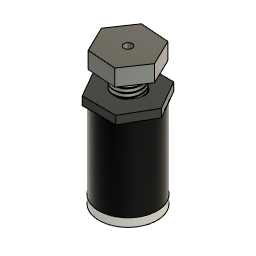
Electrode holder v2 (Autodesk Fusion 360 design; units mm, degrees)
Autodesk Fusion 360 part; units mm, degrees
note: some values were not read from the file. Set by a fixed rule: which face or edge a step refers to.
sketch "Sketch1" plane through (0, 0, 0) normal (0, 0, 1) x (1, 0, 0)
  circle A0 centre (0, 0) radius 5
  circle A1 centre (0, 0) radius 7
  dimension "d1" = 10
  dimension "d2" = 14
  constraint coincident A0.centre A1.centre
  constraint concentric A0 A1
  measures "d1" diameter of A0
  measures "d2" diameter of A1
extrude "Extrude1" add sketch "Sketch1" along normal blind 2 makes body 1
ref_plane "WorkPlane1" through (0, 0, 2.1) normal (0, 0, 1) x (1, 0, 0)
sketch "Sketch2" plane through (0, 0, 2.1) normal (0, 0, 1) x (1, 0, 0)
  circle A0 centre (0, 0) radius 5
  circle A1 centre (0, 0) radius 7
  dimension "d6" = 10
  dimension "d7" = 14
  constraint coincident A0.centre A1.centre
  constraint concentric A0 A1
  measures "d6" diameter of A0
  measures "d7" diameter of A1
extrude "Extrude2" add sketch "Sketch2" along normal blind 10 separate body makes body 2
sketch "Sketch3" plane through (0, 0, 0) normal (0, 0, -1) x (1, 0, 0)
  circle A0 centre (0, 0) radius 5
  circle A1 centre (0, 0) radius 7
  circle A2 centre (0, 0) radius 5
  circle A3 centre (0, 0) radius 4.5
  dimension "d10" = 9
  constraint coincident A0.centre A1.centre
  measures "d10" diameter of A3
extrude "Extrude3" add sketch "Sketch3" against normal blind 5.5 separate body contours A0 A2 makes body 3
combine "Combine1" operation add target body 3 tool bodies 1
sketch "Sketch4" plane through (0, 0, 12.1) normal (0, 0, 1) x (-1, 0, 0)
  circle A0 centre (0, 0) radius 5
  circle A1 centre (0, 0) radius 7
  circle A2 centre (0, 0) radius 4.5
  dimension "d13" = 9
  constraint coincident A0.centre A1.centre
  measures "d13" diameter of A2
extrude "Extrude4" add sketch "Sketch4" against normal blind 6.5 contours A0 bodies 2
sketch "Sketch5" plane through (0, 0, 12.1) normal (0, 0, 1) x (-1, 0, 0)
  circle A0 centre (0, 0) radius 4.5
  circle A1 centre (0, 0) radius 7
  line L0 (0, 0) -> (0, 4.5)
  circle A2 centre (0, 4.5) radius 1
  dimension "d16" = 2
  constraint coincident A0.centre A1.centre
  constraint coincident A0 L0.end
  constraint vertical L0
  constraint coincident L0.end A2.centre
  measures "d16" diameter of A2
extrude "Extrude5" cut sketch "Sketch5" against normal blind 8 contours A0 A2 picked at (-0.226, 4.8088) bodies 2
extrude "Extrude6" add 1 faces at (2.7671, -5.493, 12.1) along direction (0, 0, 1) blind 10 on bodies 2 bodies 2
sketch "Sketch6" plane through (0, 0, 0) normal (1, 0, 0) x (0, 1, 0)
  line L0 (-4.5, 5.5) -> (4.5, 5.5)
  line L1 (4.5, 0) -> (-4.5, 0)
  line L2 (-4.5, 0) -> (-4.5, 23.0015) construction
  circle A0 centre (-4.5, 8) radius 1
  circle A1 centre (-4.5, 12) radius 1
  circle A2 centre (-4.5, 16) radius 1
  circle A3 centre (-4.5, 20) radius 1
  dimension "d21" = 2
  dimension "d22" = 8
  dimension "d23" = 2
  dimension "d24" = 2
  dimension "d25" = 2
  dimension "d27" = 4
  dimension "d28" = 4
  dimension "d29" = 4
  constraint coincident L1.end L2.start
  constraint perpendicular L1 L2
  constraint coincident L2 A0.centre
  constraint coincident L2 A1.centre
  constraint coincident L2 A2.centre
  constraint coincident L2 A3.centre
  measures "d21" diameter of A0
  measures "d22" distance of L1.end A0.centre
  measures "d23" diameter of A1
  measures "d24" diameter of A2
  measures "d25" diameter of A3
  measures "d27" distance of A0.centre A1.centre
  measures "d28" distance of A1.centre A2.centre
  measures "d29" distance of A2.centre A3.centre
revolve "Revolve1" cut sketch "Sketch6" angle 40 about axis through (0, 0, 1.75) along (0, 0, -1) bodies 2
mirror "Mirror1" about plane through (0, 0, 0) normal (0, 1, 0) of "Extrude5"
extrude "Extrude7" cut 1 faces at (0, 5.1605, 4.1) along direction (0, 0, 1) blind 26.5 on bodies 2 bodies 2
ref_plane "WorkPlane2" through (0, 0, 12.125) normal (0.34202, 0.939693, 0) x (0, 0, 1)
mirror "Mirror2" about plane through (0, 0, 12.125) normal (0.34202, 0.939693, 0) of "Revolve1"
sketch "Sketch7" plane through (0, 0, 22.1) normal (0, 0, 1) x (-1, 0, 0)
  arc A0 (-0.9091, -4.9167) -> (0.9091, -4.9167) centre (0, -4.5) ccw
  arc A1 (0.9938, 4.3889) -> (-0.9938, 4.3889) centre (0, 4.5) ccw
  arc A2 (-0.9938, 4.3889) -> (0.9938, 4.3889) centre (0, 0) ccw
  circle A3 centre (0, 0) radius 7
  arc A4 (-0.9091, -4.9167) -> (0.9091, -4.9167) centre (0, 0) ccw
ref_plane "WorkPlane3" through (0, 0, 23.1) normal (0, 0, 1) x (-1, 0, 0)
sketch "Sketch8" plane through (0, 0, 23.1) normal (0, 0, 1) x (1, 0, 0)
  circle A0 centre (0, 0) radius 4.4
  circle A1 centre (0, 0) radius 2.5
  dimension "d40" = 8.8
  dimension "d43" = 5
  constraint coincident A0.centre A1.centre
  measures "d40" diameter of A0
  measures "d43" diameter of A1
extrude "Extrude9" add sketch "Sketch8" along normal blind 2 separate body makes body 4
sketch "Sketch9" plane through (0, 0, 0) normal (1, 0, 0) x (0, 1, 0)
  line L0 (4.4, 25.1) -> (-4.4, 25.1)
  line L1 (4.4, 23.1) -> (-4.4, 23.1)
  line L2 (-4.4, 25.1) -> (-4.4, 23.1) construction
  line L3 (4.4, 25.1) -> (4.4, 23.1) construction
  circle A0 centre (-4.4, 24.1) radius 1
  circle A1 centre (4.4, 24.1) radius 1
  line L4 (-4.4, 25.1) -> (-4.4, 23.1)
  line L5 (4.4, 25.1) -> (4.4, 23.1)
  constraint coincident L0.end L2.start
  constraint coincident L1.end L2.end
  constraint coincident L0.start L3.start
  constraint coincident L1.start L3.end
  constraint midpoint L2 A0.centre
  constraint coincident L1.end A0
  constraint midpoint L3 A1.centre
  constraint coincident L0.start A1
revolve "Revolve2" add sketch "Sketch9" angle 360 about axis through (0, 4.4, 25.1) along (0, 0, -1) contours A1 L5 picked at (4.6804, 24.2802) bodies 4
revolve "Revolve3" add sketch "Sketch9" angle 360 about axis through (0, -4.4, 25.1) along (0, 0, -1) contours A0 L4 picked at (-4.7324, 24.0751) bodies 4
extrude "Extrude10" add 1 faces at (-3.3863, -1.6307, 25.1) along direction (0, 0, 1) blind 15 on bodies 4 bodies 4
extrude "Extrude11" add 1 faces at (-3.3863, -1.6307, 23.1) along direction (0, 0, -1) blind 3 on bodies 4 bodies 4
sketch "Sketch16" plane through (0, 0, 40.1) normal (0, 0, 1) x (-1, 0, 0)
  circle A0 centre (0, 0) radius 2.5
  circle A1 centre (0, 0) radius 4.4
  line L0 (4.0415, -7) -> (8.0829, 0)
  line L1 (8.0829, 0) -> (4.0415, 7)
  line L2 (4.0415, 7) -> (-4.0415, 7)
  line L3 (-4.0415, 7) -> (-8.0829, 0)
  line L4 (-8.0829, 0) -> (-4.0415, -7)
  line L5 (-4.0415, -7) -> (4.0415, -7)
  dimension "d70" = 7
  constraint coincident A0.centre A1.centre
  measures "d70" distance of A0.centre L5
extrude "Extrude18" add sketch "Sketch16" against normal blind 2 contours L0 L1 L2 L3 L4 L5 bodies 4
thread "Thread1" "ISO Metric profile 7.0 M7x1 6H" major diameter 7.1472 minor diameter 6.0355 pitch 1 angle 60 modelled right hand crest width 0.2748 on face at (2.4876, -0.2489, 35.1) crest through (3.0178, 0, 20.35) on face at (2.4876, -0.2489, 23.7667) crest through (3.0178, 0, 20.35) on face at (2.4969, -0.1246, 21.1) crest through (3.0178, 0, 20.35) on bodies 4
ref_plane "WorkPlane4" through (0, 0, 46) normal (0, 0, 1) x (1, 0, 0)
sketch "Sketch10" plane through (0, 0, 46) normal (0, 0, 1) x (1, 0, 0)
  circle A0 centre (0, 0) radius 2.5
  circle A1 centre (0, 0) radius 1.5
  dimension "d51" = 5
  dimension "d52" = 3
  constraint coincident A0.centre A1.centre
  constraint concentric A0 A1
  measures "d51" diameter of A0
  measures "d52" diameter of A1
extrude "Extrude12" add sketch "Sketch10" along normal blind 30 separate body makes body 5
sketch "Sketch15" plane through (0, 0, 76) normal (0, 0, 1) x (-1, 0, 0)
  circle A0 centre (0, 0) radius 1.5
  circle A1 centre (0, 0) radius 2.5
  line L0 (3.0264, -6.2322) -> (6.9105, -0.4951)
  line L1 (6.9105, -0.4951) -> (3.884, 5.7371)
  line L2 (3.884, 5.7371) -> (-3.0264, 6.2322)
  line L3 (-3.0264, 6.2322) -> (-6.9105, 0.4951)
  line L4 (-6.9105, 0.4951) -> (-3.884, -5.7371)
  line L5 (-3.884, -5.7371) -> (3.0264, -6.2322)
  dimension "d65" = 6
  constraint coincident A0.centre A1.centre
  measures "d65" distance of A0.centre L5
extrude "Extrude16" add sketch "Sketch15" along normal blind 4 contours A1 | L0 L1 L2 L3 L4 L5 bodies 5
thread "Thread2" "ISO Metric profile 7.0 M7x1 6g" major diameter 6.884 minor diameter 5.744 pitch 1 angle 60 modelled right hand crest width 0.1446 on face at (2.4876, -0.2489, 66) crest through (3.442, 0, 45.75) on bodies 5
move_body "Move1" bodies 4 to x (1, 0, 0) y (0, 1, 0) z (0, 0, 1) at (0, 0, -16)
move_body "Move2" bodies 5 to x (1, 0, 0) y (0, 1, 0) z (0, 0, 1) at (0, 0, -46.9)
sketch "Sketch17" plane through (0, 0, -0.9) normal (0, 0, -1) x (1, 0, 0)
  spline S0 degree 3 poles (-1.6675, 2.3384) (-1.9957, 2.1488) (-2.2829, 1.8959) (-2.755, 1.2848) (-2.9311, 0.9293) (-3.1433, 0.1579) (-3.1723, -0.2519) (-3.0724, -1.0738) (-2.9393, -1.4773) (-2.5912, -2.0994) (-2.4153, -2.334) (-2.0032, -2.7562) (-1.7674, -2.9409) (-1.5108, -3.0927) knots 0 0 0 0 0.1137 0.1137 0.231484 0.231484 0.35335 0.35335 0.479296 0.479296 0.566597 0.566597 0.655752 0.655752 0.655752 0.655752
  arc A0 (-1.5108, -3.0927) -> (1.5108, -3.0927) centre (0, 0) ccw
  spline S1 degree 3 poles (1.5108, -3.0927) (1.8895, -2.8686) (2.2216, -2.5737) (2.7435, -1.8828) (2.9326, -1.4966) (3.146, -0.6861) (3.1733, -0.2711) (3.0667, 0.5321) (2.9389, 0.9131) (2.6109, 1.4838) (2.4525, 1.6916) (2.0894, 2.0556) (1.8874, 2.2114) (1.6675, 2.3384) knots 0 0 0 0 0.132024 0.132024 0.259957 0.259957 0.383795 0.383795 0.503539 0.503539 0.581826 0.581826 0.658261 0.658261 0.658261 0.658261
  arc A1 (1.6675, 2.3384) -> (-1.6675, 2.3384) centre (0, 0) ccw
  circle A2 centre (0, 0) radius 1.5
  circle A3 centre (0, 0) radius 1
  dimension "d73" = 2
  constraint coincident A0.centre A1.centre
  measures "d73" diameter of A3
extrude "Extrude19" add sketch "Sketch17" against normal blind 34 contours A2 bodies 5
thread "Thread3" "ISO Metric profile 12.0 M12x1.75 6g" major diameter 11.8335 minor diameter 9.8365 pitch 1.75 angle 60 modelled right hand crest width 0.2518 on face at (4.9752, -0.4978, 3.1667) crest through (5.9168, 0, 1.5625) on bodies 3
thread "Thread4" "ISO Metric profile 12.0 M12x1.75 6H" major diameter 12.2265 minor diameter 10.2735 pitch 1.75 angle 60 modelled right hand crest width 0.4769 on face at (-1.4549, -4.7836, 3.9333) crest through (5.1368, 0, 2.5375) on bodies 2
move_body "Move3" bodies 3 to x (1, 0, 0) y (0, 1, 0) z (0, 0, 1) at (0, 0, 0.1)
move_body "Move4" bodies 4 to x (1, 0, 0) y (0, 1, 0) z (0, 0, 1) at (0, 0, 0)
sketch "Sketch18" plane through (0, 0, 33.1) normal (0, 0, 1) x (-1, 0, 0)
  circle A0 centre (0, 0) radius 1
  line L0 (-3.884, -5.7371) -> (3.0264, -6.2322)
  line L1 (3.0264, -6.2322) -> (6.9105, -0.4951)
  line L2 (6.9105, -0.4951) -> (3.884, 5.7371)
  line L3 (3.884, 5.7371) -> (-3.0264, 6.2322)
  line L4 (-3.0264, 6.2322) -> (-6.9105, 0.4951)
  line L5 (-6.9105, 0.4951) -> (-3.884, -5.7371)
  line L6 (0, 0) -> (-17.0369, 0)
  line L7 (-17.0369, 0) -> (-17.0369, -15.2058)
  line L8 (-17.0369, -15.2058) -> (0, -15.2058)
  line L9 (0, -15.2058) -> (0, 0)
  line L10 (0, 0) -> (-17.0369, 0)
  line L11 (-17.0369, 0) -> (-17.0369, 15.2148)
  line L12 (-17.0369, 15.2148) -> (0, 15.2148)
  line L13 (0, 15.2148) -> (0, 0)
  constraint horizontal L6
  constraint vertical L7
  constraint horizontal L8
  constraint vertical L9
  constraint coincident A0.centre L6.start
  constraint horizontal L10
  constraint vertical L11
  constraint horizontal L12
  constraint vertical L13
